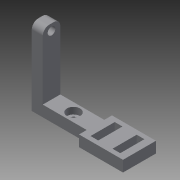
# Autodesk Inventor part: switch bracket v5.1
Saved by Autodesk Inventor 2013 SP2 (Build 170200200, 200)
## iProperties
Created: 2018-01-16
Part Number: switch bracket v5.1
Material: Generic
Document SubType Name: Modeling
Designer: hdv
Density: 1 g/cm^3
Author: hdv
Autodesk Inventor part; units mm, degrees
ref_plane "YZ Plane" through (0, 0, 0) normal (1, 0, 0) x (0, 1, 0)
ref_plane "XZ Plane" through (0, 0, 0) normal (0, 1, 0) x (-1, 0, 0)
ref_plane "XY Plane" through (0, 0, 0) normal (0, 0, 1) x (1, 0, 0)
sketch "Sketch1" plane through (0, 0, 0) normal (0, 0, 1) x (1, 0, 0)
  line L0 (0, 15) -> (20, 15)
  line L1 (20, 15) -> (20, 0)
  line L2 (20, 0) -> (0, 0)
  line L3 (0, 0) -> (0, 15)
  line L4 (3.25, 13) -> (6.75, 13)
  line L5 (6.75, 13) -> (6.75, 2)
  line L6 (6.75, 2) -> (3.25, 2)
  line L7 (3.25, 2) -> (3.25, 13)
  line L8 (13.25, 13) -> (16.75, 13)
  line L9 (16.75, 13) -> (16.75, 2)
  line L10 (16.75, 2) -> (13.25, 2)
  line L11 (13.25, 2) -> (13.25, 13)
  line L12 (0, 11.5) -> (-25, 11.5)
  line L13 (-25, 11.5) -> (-25, 3.5)
  line L14 (-25, 3.5) -> (0, 3.5)
  line L15 (0, 3.5) -> (0, 11.5)
  circle A0 centre (-10, 7.5) radius 1.75
  point P0 (0, -23)
  point P1 (0, 7.5)
  dimension "d0" = 20
  dimension "d1" = 2
  dimension "d2" = 2
  dimension "d3" = 3.5
  dimension "d4" = 3.25
  dimension "d5" = 6.5
  dimension "d6" = 3.5
  dimension "d8" = 15
  dimension "d9" = 25
  dimension "d10" = 8
  dimension "d22" = 3.5
  dimension "d23" = 10
  constraints: 32 end point, 8 parallel, 4 horizontal, 4 perpendicular, 2 collinear, 2 midpoint, 1 centre point, 1 coincident, 1 horizontal alignment, 1 point on line
  measures "d0" distance of L0.start L0.end
  measures "d1" distance between parallel lines of L8 L0
  measures "d2" distance between parallel lines of L2 L10
  measures "d3" distance of L9.end L10.end
  measures "d4" distance between parallel lines of L9 L1
  measures "d5" distance between parallel lines of L5 L11
  measures "d6" distance of L5.end L6.end
  measures "d8" distance of L2.end L0.start
  measures "d9" distance of L14.end L13.end
  measures "d10" distance of L13.end L12.end
  measures "d22" diameter of A0
  measures "d23" distance from line of A0.centre L15
extrude "Extrusion1" add sketch "Sketch1" along normal blind 5
sketch "Sketch2" plane through (0, 0, 5) normal (0, 0, 1) x (1, 0, 0)
  line L0 (-25, 3.5) -> (0, 3.5) projected
  line L1 (-25, 11.5) -> (-20, 11.5)
  line L2 (-20, 11.5) -> (-20, 3.5)
  line L3 (-20, 3.5) -> (-25, 3.5)
  line L4 (-25, 3.5) -> (-25, 11.5)
  dimension "d24" = 5
  constraints: 8 end point, 2 parallel, 1 horizontal, 1 perpendicular, 1 point on line
  measures "d24" distance between parallel lines of L4 L2
extrude "Extrusion2" add sketch "Sketch2" along normal blind 30
sketch "Sketch3" plane through (-25, 3.5, 0) normal (-1, 0, 0) x (0, 0, 1)
  line L0 (35, 8) -> (35, 0) projected
  circle A0 centre (32, 4) radius 1.75
  point P0 (0, -3.5)
  point P1 (35, 4)
  dimension "d17" = 3.5
  dimension "d18" = 3
  constraints: 1 centre point, 1 horizontal alignment, 1 midpoint
  measures "d17" diameter of A0
  measures "d18" distance from line of A0.centre L0
extrude "Extrusion3" cut sketch "Sketch3" against normal blind 35
fillet "Fillet1" radius 3 2 edges at (-22.5, 11.5, 35) (-22.5, 3.5, 35)
sketch "Sketch4" plane through (0, 0, 5) normal (0, 0, 1) x (1, 0, 0)
  circle A0 centre (-10, 7.5) radius 1.75 projected
  circle A1 centre (-10, 7.5) radius 3
  dimension "d26" = 6
  constraints: 1 centre point, 1 coincident
  measures "d26" diameter of A1
extrude "Extrusion4" cut sketch "Sketch4" against normal blind 3
equation "\"d2\" = d1"
equation "\"d6\" = d3"
body "Solid1"
